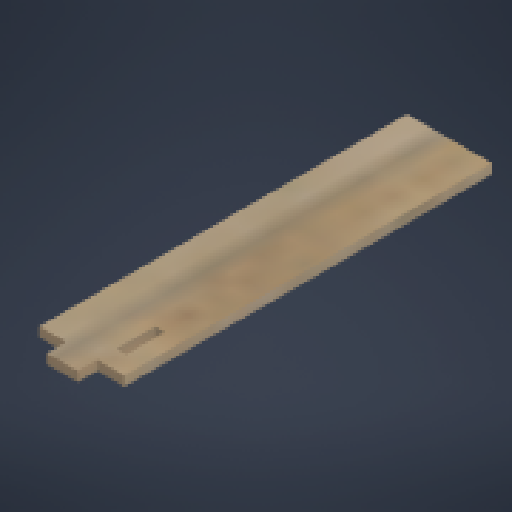
# Autodesk Inventor part: dish_upper
Saved by Autodesk Inventor 2026.1 (Build 301233020, 233B)
## iProperties
Created: 2025-09-27
Part Number: dish_upper
Material: 木材 (カエデ材)
Document SubType Name: モデリング
Designer: hibik
Density: 0.67 g/cm^3
Appearance: ナチュラル カエデ材 - 光沢 濃い着色
Author: hibik
Autodesk Inventor part; units mm, degrees
ref_plane "YZ Plane" through (0, 0, 0) normal (1, 0, 0) x (0, 1, 0)
ref_plane "XZ Plane" through (0, 0, 0) normal (0, 1, 0) x (-1, 0, 0)
ref_plane "XY Plane" through (0, 0, 0) normal (0, 0, 1) x (1, 0, 0)
sketch "スケッチ1" plane through (0, 0, 0) normal (0, 1, 0) x (-1, 0, 0)
  line L0 (11, 11) -> (-11, 11)
  line L1 (-11, 11) -> (-11, -9.8801)
  line L2 (11, -9) -> (11, 11)
  line L3 (-11, -5.4423) -> (-11, -109)
  line L4 (-11, -109) -> (11, -109)
  line L5 (11, -109) -> (11, -9)
  circle A0 centre (0, 0) radius 11
  point P0 (11, 1)
  dimension "d1" = 20
  dimension "d12" = 22
  dimension "d13" = 120
  constraints: 12 end point, 3 tangent, 2 parallel, 1 centre point, 1 collinear, 1 horizontal, 1 midpoint, 1 perpendicular
  measures "d1" distance of L2.start L0.start
  measures "d12" diameter of A0
  measures "d13" distance between parallel lines of L4 L0
extrude "押し出し1" add sketch "スケッチ1" along normal blind 2.5
sketch "スケッチ2" plane through (0, 0, 0) normal (0, -1, 0) x (1, 0, 0)
  line L0 (11, 11) -> (-11, 11)
  line L1 (-11, 11) -> (-11, -14)
  line L2 (-11, -14) -> (11, -14)
  line L3 (11, -14) -> (11, 11)
  line L4 (4, -14) -> (-4, -14)
  line L5 (-4, -14) -> (-4, -9)
  line L6 (-4, -9) -> (4, -9)
  line L7 (4, -9) -> (4, -14)
  point P0 (0, 0)
  point P1 (0, -14)
  dimension "d14" = 25
  dimension "d15" = 8
  dimension "d16" = 5
  constraints: 16 end point, 4 parallel, 2 coincident, 2 horizontal, 2 midpoint, 2 perpendicular, 1 point on line
  measures "d14" distance of L2.end L0.start
  measures "d15" distance of L5.end L6.end
  measures "d16" distance of L6.end L4.start
extrude "押し出し2" cut sketch "スケッチ2" against normal through all contours L3 L2 L7 L6 L5 L1 L0
sketch "スケッチ3" plane through (0, 2.5, 0) normal (0, 1, 0) x (1, 0, 0)
  line L0 (4, 19) -> (6.5, 19)
  line L1 (6.5, 19) -> (6.5, 29)
  line L2 (6.5, 29) -> (4, 29)
  line L3 (4, 29) -> (4, 19)
  line L4 (4, 14) -> (11, 14) projected
  line L5 (4, 9) -> (4, 14) projected
  point P0 (0, 0)
  dimension "d19" = 2.5
  dimension "d20" = 10
  dimension "d21" = 5
  constraints: 8 end point, 2 parallel, 1 collinear, 1 horizontal, 1 perpendicular
  measures "d19" distance of L0.start L0.end
  measures "d20" distance of L0.end L1.end
  measures "d21" distance between parallel lines of L4 L0
extrude "押し出し3" cut sketch "スケッチ3" against normal through all
equation "\"BendRadius\" = Thickness"
equation "\"BendReliefWidth\" = Thickness"
equation "\"BendReliefDepth\" = 0.5 * Thickness"
equation "\"CornerReliefSize\" = 4 * Thickness"
equation "\"MinimumRemnant\" = 2 * Thickness"
equation "\"TransitionRadius\" = BendRadius"
equation "\"JacobiRadiusSize\" = BendRadius"
equation "\"GapSize\" = Thickness"
equation "\"Thickness\" = 3.048"
